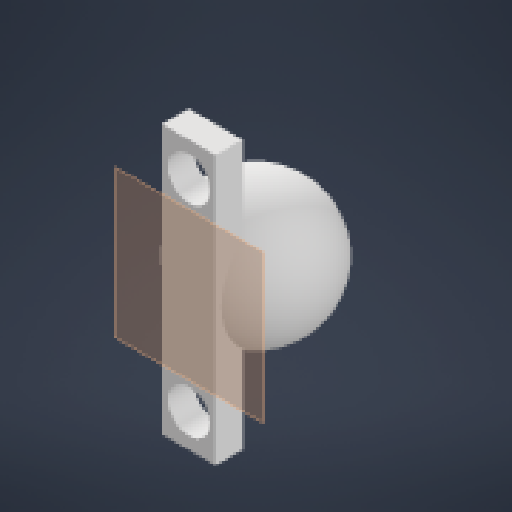
# Autodesk Inventor part: Rueda trasera
Saved by Autodesk Inventor 2023 (Build 270158000, 158)
## iProperties
Created: 2019-04-01
Part Number: Rueda trasera
Material: Genérico
Document SubType Name: Modeling
Designer: Marcelo
Density: 1 g/cm^3
Appearance: Valor por defecto
Author: Marcelo
Autodesk Inventor part; units mm, degrees
ref_plane "YZ Plane" through (0, 0, 0) normal (1, 0, 0) x (0, 1, 0)
ref_plane "XZ Plane" through (0, 0, 0) normal (0, 1, 0) x (-1, 0, 0)
sketch "Boceto1" plane through (0, 0, 0) normal (0, 0, 1) x (1, 0, 0)
  arc A0 (0, 5) -> (0, -5) centre (0, 0) ccw
  line L0 (0, 5) -> (0, -5)
  constraints: 2 end point, 2 point on circle, 1 centre point, 1 coincident, 1 vertical
revolve "Revolución1" add sketch "Boceto1" angle 360 about axis through (0, 5, 0) along (0, -1, 0)
ref_plane "Plano de trabajo1" through (0, 0, 5) normal (0, 0, 1) x (1, 0, 0)
sketch "Boceto2" plane through (0, 0, 5) normal (0, 0, 1) x (1, 0, 0)
  line L0 (-2, -10) -> (2, -10)
  line L1 (2, -10) -> (2, 10)
  line L2 (2, 10) -> (-2, 10)
  line L3 (-2, 10) -> (-2, -10)
  line L4 (-2, -10) -> (2, 10) construction
  line L5 (2, -10) -> (-2, 10) construction
  point P0 (0, 0)
  dimension "d3" = 4
  dimension "d4" = 20
  constraints: 12 end point, 2 equal length, 2 midpoint, 1 parallel, 1 vertical
  measures "d3" distance of L2.end L1.end
  measures "d4" distance of L1.end L0.end
extrude "Extrusión1" add sketch "Boceto2" against normal blind 2
sketch "Boceto3" plane through (0, 0, 5) normal (0, 0, 1) x (1, 0, 0)
  point P0 (0, 0)
  point P1 (0, 7.5)
  point P2 (0, -7.5)
hole "Agujero1" at (0, 7.5, 5) at (0, -7.5, 5) direction (0, 0, -1) diameter 3.175 end through all
